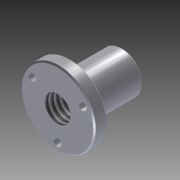
# Autodesk Inventor part: ZACMENut
Saved by Autodesk Inventor 2015 SP1 (Build 190203100, 203)
## iProperties
Created: 2014-01-02
Part Number: ZACMENut
Material: ABS Plastic
Document SubType Name: Modeling
Designer: Jack
Density: 1.06 g/cm^3
Appearance: Smooth - White
Mass: 5.32083 g
Surface Area: 33.614 cm^2
Volume: 5.01965 cm^3
Author: Jack
Autodesk Inventor part; units mm, degrees
ref_plane "YZ Plane" through (0, 0, 0) normal (1, 0, 0) x (0, 1, 0)
ref_plane "XZ Plane" through (0, 0, 0) normal (0, 1, 0) x (-1, 0, 0)
ref_plane "XY Plane" through (0, 0, 0) normal (0, 0, 1) x (1, 0, 0)
sketch "Sketch1" plane through (0, 0, 0) normal (0, 1, 0) x (-1, 0, 0)
  circle A0 centre (0, 0) radius 14.25
  dimension "d0" = 28.5
  constraints: 1 centre point, 1 coincident
  measures "d0" diameter of A0
extrude "Extrusion1" add sketch "Sketch1" along normal blind 5
sketch "Sketch2" plane through (0, 5, 0) normal (0, 1, 0) x (1, 0, 0)
  circle A0 centre (0, 0) radius 14.25 projected
  circle A1 centre (0, 0) radius 7.9
  dimension "d3" = 15.8
  constraints: 1 centre point, 1 coincident
  measures "d3" diameter of A1
extrude "Extrusion2" add sketch "Sketch2" along normal blind 20 contours A1
sketch "Sketch3" plane through (0, 25, 0) normal (0, 1, 0) x (1, 0, 0)
  circle A0 centre (0, 0) radius 7.9 projected
  circle A1 centre (0, 0) radius 5
  dimension "d6" = 10
  constraints: 1 centre point, 1 coincident
  measures "d6" diameter of A1
extrude "Extrusion3" cut sketch "Sketch3" against normal blind 25.6 contours A1
chamfer "Chamfer1" distance 0.5 angle 45 1 edges at (-7.9, 25, 0)
chamfer "Chamfer2" distance 0.5 angle 45 3 edges at (-7.9, 5, 0) (14.25, 5, 0) (14.25, 0, 0)
thread "Thread1" size "TR10x2" class "7H" standard "ISO Metric Trapezoidal Threads" full length
sketch "Sketch4" plane through (0, 0, 0) normal (0, -1, 0) x (1, 0, 0)
  circle A0 centre (0, 0) radius 13.75 projected
  line L0 (0, 0) -> (0, -13.75) construction
  line L1 (0, 0) -> (-11.9078, 6.875) construction
  line L2 (0, 0) -> (11.9078, 6.875) construction
  circle A1 centre (0, 0) radius 14.25 projected
  circle A2 centre (0, 0) radius 11.25 construction
  circle A3 centre (9.7428, 5.625) radius 1.5
  circle A4 centre (0, -11.25) radius 1.5
  circle A5 centre (-9.7428, 5.625) radius 1.5
  dimension "d17" = 120
  dimension "d18" = 120
  dimension "d22" = 22.5
  dimension "d23" = 3
  dimension "d24" = 3
  dimension "d25" = 3
  constraints: 6 end point, 6 point on circle, 4 centre point, 3 point on line, 1 coincident, 1 vertical
  measures "d17" angle of L0 L1
  measures "d18" angle of L2 L0
  measures "d22" diameter of A2
  measures "d23" diameter of A3
  measures "d24" diameter of A4
  measures "d25" diameter of A5
extrude "Extrusion4" cut sketch "Sketch4" against normal blind 5 contours A3 | A4 | A5
body "Solid1"
